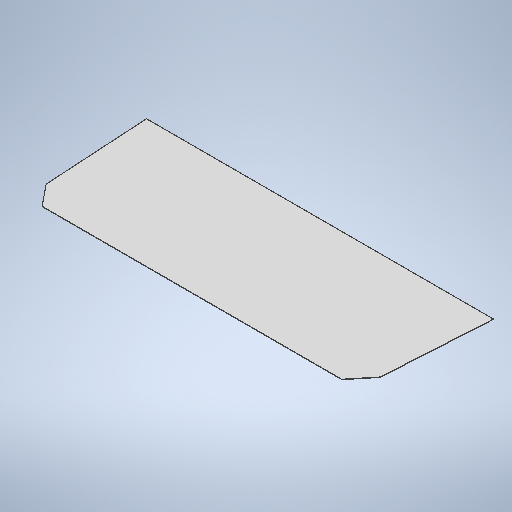
# Autodesk Inventor part: MSC 075 face 2
Saved by Autodesk Inventor 2025 (Build 290162010, 162A)
## iProperties
Created: 2024-06-16
Part Number: MSC 075 face 2
Material: AISI304
Document SubType Name: Sheet Metal
Designer: admin
Density: 8 g/cm^3
Sheet Metal Rule: AISI304 2mm Die16
Appearance: Default
Stock Number: МОО 075 морда 2
Flat Pattern Width: 58.4545 cm
Flat Pattern Length: 158.425 cm
Flat Pattern Area: 9260.67 cm^2
Sheet Metal Width: 584,545 mm
Sheet Metal Length: 1584,253 mm
Sheet Metal Area: 926067,212 mm^2
Author: admin
Autodesk Inventor part; units mm, degrees
ref_plane "YZ Plane" through (0, 0, 0) normal (1, 0, 0) x (0, 1, 0)
ref_plane "XZ Plane" through (0, 0, 0) normal (0, 1, 0) x (-1, 0, 0)
ref_plane "XY Plane" through (0, 0, 0) normal (0, 0, 1) x (1, 0, 0)
sketch "Sketch1" plane through (0, 0, 0) normal (0, 0, 1) x (1, 0, 0)
  line L0 (792.1263, 0) -> (792.1263, -584.5451) construction
  line L1 (792.1263, -584.5451) -> (0, -584.5451)
  line L2 (751.2327, -486.2569) -> (671.2185, -584.5451) construction
  ellipse E0 centre (-10250, 888.2841) end of major axis (-10250, -13540.3827) minor radius 11053 (753.0938, -481.2962) -> (781.7614, -5.752) ccw construction
  line L3 (792.1263, 0) -> (762.7078, -488.0006)
  line L4 (684.1131, -584.5451) -> (792.1263, -451.8633)
  line L5 (753.0938, -481.2962) -> (763.0757, -481.898) construction
  line L6 (781.7614, -5.752) -> (791.7433, -6.3537) construction
  line L7 (0, -584.5451) -> (0, 0)
  line L8 (0, 0) -> (792.1263, 0)
  dimension "d3" = 10
  dimension "d4" = 10
  dimension "d5" = 10
  measures "d3" distance between parallel lines of L4 L2
  measures "d4" distance of L5.start L5.end
  measures "d5" distance of L6.start L6.end
extrude "Plate1" add sketch "Sketch1" along normal blind 2
mirror "Mirror1" about plane through (0, 0, 0) normal (1, 0, 0) of "Plate1"
equation "\"d2\" = Thickness"
equation "\"BendReliefWidth\" = Thickness"
equation "\"BendReliefDepth\" = 0.5 * Thickness"
equation "\"CornerReliefSize\" = 4 * Thickness"
equation "\"MinimumRemnant\" = 2 * Thickness"
equation "\"TransitionRadius\" = BendRadius"
equation "\"JacobiRadiusSize\" = BendRadius"
equation "\"GapSize\" = Thickness"
equation "\"Thickness\" = 2"
equation "\"BendRadius\" = 2.75"
body "Solid1"
